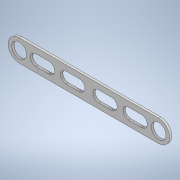
# Autodesk Inventor part: p1
Saved by Autodesk Inventor 2022 (Build 260153000, 153)
## iProperties
Created: 2022-03-17
Part Number: p1
Material: Generic
Document SubType Name: Modeling
Designer: br4ch
Density: 1 g/cm^3
Appearance: Default
Author: br4ch
Autodesk Inventor part; units mm, degrees
ref_plane "YZ Plane" through (0, 0, 0) normal (1, 0, 0) x (0, 1, 0)
ref_plane "XZ Plane" through (0, 0, 0) normal (0, 1, 0) x (-1, 0, 0)
ref_plane "XY Plane" through (0, 0, 0) normal (0, 0, 1) x (1, 0, 0)
sketch "Sketch2" plane through (0, 0, 0) normal (0, 0, 1) x (1, 0, 0)
  line L0 (-108, -20.3137) -> (82, -20.3137) construction
  line L1 (-108, -35.3137) -> (82, -35.3137)
  line L2 (82, -5.3137) -> (-108, -5.3137)
  arc A0 (-108, -5.3137) -> (-108, -35.3137) centre (-108, -20.3137) ccw
  arc A1 (82, -35.3137) -> (82, -5.3137) centre (82, -20.3137) ccw
  circle A2 centre (-108, -20.3137) radius 10
  circle A3 centre (82, -20.3137) radius 10
  line L3 (-85, -20.3137) -> (-67, -20.3137) construction
  line L4 (-85, -27.8137) -> (-67, -27.8137)
  line L5 (-67, -12.8137) -> (-85, -12.8137)
  arc A4 (-85, -12.8137) -> (-85, -27.8137) centre (-85, -20.3137) ccw
  arc A5 (-67, -27.8137) -> (-67, -12.8137) centre (-67, -20.3137) ccw
  line L6 (-13, -46) -> (-13, 6) construction
  arc A6 (-26, -27.8137) -> (-26, -12.8137) centre (-26, -20.3137) ccw
  line L7 (-44, -20.3137) -> (-26, -20.3137) construction
  line L8 (-44, -27.8137) -> (-26, -27.8137)
  line L9 (-26, -12.8137) -> (-44, -12.8137)
  arc A7 (-44, -12.8137) -> (-44, -27.8137) centre (-44, -20.3137) ccw
  line L10 (59, -20.3137) -> (41, -20.3137) construction
  line L11 (59, -27.8137) -> (41, -27.8137)
  line L12 (41, -12.8137) -> (59, -12.8137)
  arc A8 (59, -27.8137) -> (59, -12.8137) centre (59, -20.3137) ccw
  arc A9 (41, -12.8137) -> (41, -27.8137) centre (41, -20.3137) ccw
  arc A10 (0, -12.8137) -> (0, -27.8137) centre (0, -20.3137) ccw
  line L13 (18, -20.3137) -> (0, -20.3137) construction
  line L14 (18, -27.8137) -> (0, -27.8137)
  line L15 (0, -12.8137) -> (18, -12.8137)
  arc A11 (18, -27.8137) -> (18, -12.8137) centre (18, -20.3137) ccw
  point P0 (0, 0)
  point P1 (-13, -20.3137)
  point P2 (-76, -20.3137)
  point P3 (-35, -20.3137)
  point P4 (50, -20.3137)
  point P5 (9, -20.3137)
  dimension "d27" = 190
  dimension "d28" = 30
  dimension "d29" = 20
  dimension "d30" = 20
  dimension "d31" = 18
  dimension "d32" = 15
  dimension "d43" = 41
  dimension "d48" = 41
  constraints: 42 end point, 20 point on circle, 14 symmetric about line, 12 centre point, 8 tangent, 3 point on line, 2 coincident, 2 horizontal, 2 midpoint, 2 parallel, 1 vertical, 16 other
  measures "d27" distance of L0.start L0.end
  measures "d28" diameter of A1
  measures "d29" diameter of A2
  measures "d30" diameter of A3
  measures "d31" distance of L3.start L3.end
  measures "d32" diameter of A5
  measures "d43" distance of L3.end L7.end
  measures "d48" distance of L3.end L0.start
extrude "Extrusion2" add sketch "Sketch2" along normal blind 3
body "Solid2"
